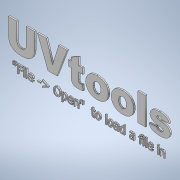
# Autodesk Inventor part: UVtools_demo_file
Saved by Autodesk Inventor 2021 (Build 250183000, 183)
## iProperties
Created: 2020-10-14
Part Number: UVtools_demo_file
Material: Generic
Document SubType Name: Modeling
Designer: tiago
Density: 1 g/cm^3
Appearance: Default
Author: tiago
## iProperties of the stored document _3DPrint.ipt
Created: 2020-10-14
Part Number: _3DPrint
Material: Generic
Document SubType Name: Modeling
Designer: tiago
Density: 1 g/cm^3
Appearance: Default
Author: tiago
Autodesk Inventor part; units mm, degrees
ref_plane "YZ Plane" through (0, 0, 0) normal (1, 0, 0) x (0, 1, 0)
ref_plane "XZ Plane" through (0, 0, 0) normal (0, 1, 0) x (-1, 0, 0)
ref_plane "XY Plane" through (0, 0, 0) normal (0, 0, 1) x (1, 0, 0)
sketch "Sketch1" plane through (0, 0, 0) normal (0, 0, 1) x (1, 0, 0)
  line L0 (-61.4135, 29.5284) -> (63.6527, 29.5284) construction
  line L1 (63.6527, 29.5284) -> (63.6527, 8.7715) construction
  line L2 (63.6527, 8.7715) -> (-61.4135, 8.7715) construction
  line L3 (-61.4135, 8.7715) -> (-61.4135, 29.5284) construction
  line L4 (-61.4135, 8.7715) -> (63.6527, 8.7715) construction
  line L5 (63.6527, 8.7715) -> (63.6527, -11.4157) construction
  line L6 (63.6527, -11.4157) -> (-61.4135, -11.4157) construction
  line L7 (-61.4135, -11.4157) -> (-61.4135, 8.7715) construction
  line L8 (-44.3664, 29.3232) -> (-38.2067, 29.3232)
  line L9 (-38.2067, 29.3232) -> (-38.2067, 17.4079)
  spline S0 degree 2 poles (-38.2067, 17.4079) (-38.2067, 15.6369) (-39.3039, 12.4801) (-41.6716, 10.1316) (-42.9805, 9.6504) knots 0 0 0 1 2 3 3 3
  spline S1 degree 2 poles (-42.9805, 9.6504) (-44.7707, 8.9767) (-47.3116, 8.9767) knots 0 0 0 1 1 1
  spline S2 degree 2 poles (-47.3116, 8.9767) (-48.7745, 8.9767) (-52.2202, 9.3809) (-54.5493, 10.5936) (-56.4742, 12.8265) (-56.8207, 14.02) knots 0 0 0 1 2 3 4 4 4
  spline S3 degree 2 poles (-56.8207, 14.02) (-57.3982, 15.9257) (-57.3982, 17.4079) knots 0 0 0 1 1 1
  line L10 (-57.3982, 17.4079) -> (-57.3982, 29.3232)
  line L11 (-57.3982, 29.3232) -> (-51.2384, 29.3232)
  line L12 (-51.2384, 29.3232) -> (-51.2384, 17.1191)
  spline S4 degree 2 poles (-51.2384, 17.1191) (-51.2384, 15.4829) (-49.4098, 13.635) (-47.7928, 13.635) knots 0 0 0 1 2 2 2
  spline S5 degree 2 poles (-47.7928, 13.635) (-46.1951, 13.635) (-44.3664, 15.4444) (-44.3664, 17.1191) knots 0 0 0 1 2 2 2
  line L13 (-44.3664, 17.1191) -> (-44.3664, 29.3232)
  line L14 (-36.1085, 29.3232) -> (-29.6408, 29.3232)
  line L15 (-29.6408, 29.3232) -> (-25.1172, 14.9247)
  line L16 (-25.1172, 14.9247) -> (-20.6898, 29.3232)
  line L17 (-20.6898, 29.3232) -> (-14.4146, 29.3232)
  line L18 (-14.4146, 29.3232) -> (-21.8448, 9.3232)
  line L19 (-21.8448, 9.3232) -> (-28.5435, 9.3232)
  line L20 (-28.5435, 9.3232) -> (-36.1085, 29.3232)
  line L21 (-6.0411, 29.3232) -> (-6.0411, 23.8179)
  line L22 (-6.0411, 23.8179) -> (-2.9805, 23.8179)
  line L23 (-2.9805, 23.8179) -> (-2.9805, 19.7563)
  line L24 (-2.9805, 19.7563) -> (-6.0411, 19.7563)
  line L25 (-6.0411, 19.7563) -> (-6.0411, 14.6167)
  spline S6 degree 2 poles (-6.0411, 14.6167) (-6.0411, 13.6928) (-5.8679, 13.3848) knots 0 0 0 1 1 1
  spline S7 degree 2 poles (-5.8679, 13.3848) (-5.5984, 12.9228) (-4.9054, 12.9228) knots 0 0 0 1 1 1
  spline S8 degree 2 poles (-4.9054, 12.9228) (-4.2895, 12.9228) (-3.1922, 13.2693) knots 0 0 0 1 1 1
  line L26 (-3.1922, 13.2693) -> (-2.788, 9.4387)
  spline S9 degree 2 poles (-2.788, 9.4387) (-4.8477, 8.9959) (-6.6379, 8.9959) knots 0 0 0 1 1 1
  spline S10 degree 2 poles (-6.6379, 8.9959) (-8.6975, 8.9959) (-10.661, 10.0546) (-11.6042, 12.2298) (-11.6042, 14.6552) knots 0 0 0 1 2 3 3 3
  line L27 (-11.6042, 14.6552) -> (-11.6042, 19.7563)
  line L28 (-11.6042, 19.7563) -> (-13.6446, 19.7563)
  line L29 (-13.6446, 19.7563) -> (-13.6446, 23.8179)
  line L30 (-13.6446, 23.8179) -> (-11.6042, 23.8179)
  line L31 (-11.6042, 23.8179) -> (-11.6042, 26.4743)
  line L32 (-11.6042, 26.4743) -> (-6.0411, 29.3232)
  spline S11 degree 2 poles (-0.9978, 16.5224) (-0.9978, 19.8525) (3.468, 24.1451) (7.2794, 24.1451) knots 0 0 0 1 2 2 2
  spline S12 degree 2 poles (7.2794, 24.1451) (11.6297, 24.1451) (13.8434, 21.6235) knots 0 0 0 1 1 1
  spline S13 degree 2 poles (13.8434, 21.6235) (15.6336, 19.583) (15.6336, 16.6187) knots 0 0 0 1 1 1
  spline S14 degree 2 poles (15.6336, 16.6187) (15.6336, 13.2693) (11.2062, 8.9959) (7.2986, 8.9959) knots 0 0 0 1 2 2 2
  spline S15 degree 2 poles (7.2986, 8.9959) (3.7952, 8.9959) (1.6393, 10.7669) knots 0 0 0 1 1 1
  spline S16 degree 2 poles (1.6393, 10.7669) (-0.9978, 12.9613) (-0.9978, 16.5224) knots 0 0 0 1 1 1
  spline S17 degree 2 poles (4.5652, 16.5417) (4.5652, 14.5975) (6.1244, 12.7495) (7.3179, 12.7495) knots 0 0 0 1 2 2 2
  spline S18 degree 2 poles (7.3179, 12.7495) (8.5113, 12.7495) (10.0513, 14.5782) (10.0513, 16.5994) knots 0 0 0 1 2 2 2
  spline S19 degree 2 poles (10.0513, 16.5994) (10.0513, 18.4666) (8.4921, 20.3145) (7.3564, 20.3145) knots 0 0 0 1 2 2 2
  spline S20 degree 2 poles (7.3564, 20.3145) (6.1437, 20.3145) (4.5652, 18.4473) (4.5652, 16.5417) knots 0 0 0 1 2 2 2
  spline S21 degree 2 poles (17.6547, 16.5224) (17.6547, 19.8525) (22.1206, 24.1451) (25.9319, 24.1451) knots 0 0 0 1 2 2 2
  spline S22 degree 2 poles (25.9319, 24.1451) (30.2823, 24.1451) (32.4959, 21.6235) knots 0 0 0 1 1 1
  spline S23 degree 2 poles (32.4959, 21.6235) (34.2861, 19.583) (34.2861, 16.6187) knots 0 0 0 1 1 1
  spline S24 degree 2 poles (34.2861, 16.6187) (34.2861, 13.2693) (29.8588, 8.9959) (25.9512, 8.9959) knots 0 0 0 1 2 2 2
  spline S25 degree 2 poles (25.9512, 8.9959) (22.4478, 8.9959) (20.2919, 10.7669) knots 0 0 0 1 1 1
  spline S26 degree 2 poles (20.2919, 10.7669) (17.6547, 12.9613) (17.6547, 16.5224) knots 0 0 0 1 1 1
  spline S27 degree 2 poles (23.2178, 16.5417) (23.2178, 14.5975) (24.777, 12.7495) (25.9704, 12.7495) knots 0 0 0 1 2 2 2
  spline S28 degree 2 poles (25.9704, 12.7495) (27.1639, 12.7495) (28.7038, 14.5782) (28.7038, 16.5994) knots 0 0 0 1 2 2 2
  spline S29 degree 2 poles (28.7038, 16.5994) (28.7038, 18.4666) (27.1446, 20.3145) (26.0089, 20.3145) knots 0 0 0 1 2 2 2
  spline S30 degree 2 poles (26.0089, 20.3145) (24.7962, 20.3145) (23.2178, 18.4473) (23.2178, 16.5417) knots 0 0 0 1 2 2 2
  line L33 (37.1735, 29.3232) -> (42.7365, 29.3232)
  line L34 (42.7365, 29.3232) -> (42.7365, 9.3232)
  line L35 (42.7365, 9.3232) -> (37.1735, 9.3232)
  line L36 (37.1735, 9.3232) -> (37.1735, 29.3232)
  line L37 (45.3159, 13.3463) -> (50.8212, 13.866)
  spline S31 degree 2 poles (50.8212, 13.866) (51.1677, 12.8843) (52.3997, 12.0373) (53.4199, 12.0373) knots 0 0 0 1 2 2 2
  spline S32 degree 2 poles (53.4199, 12.0373) (54.5556, 12.0373) (55.1716, 12.5186) knots 0 0 0 1 1 1
  spline S33 degree 2 poles (55.1716, 12.5186) (55.6528, 12.865) (55.6528, 13.404) knots 0 0 0 1 1 1
  spline S34 degree 2 poles (55.6528, 13.404) (55.6528, 14.0008) (55.0176, 14.328) knots 0 0 0 1 1 1
  spline S35 degree 2 poles (55.0176, 14.328) (54.5556, 14.559) (52.6307, 14.9055) knots 0 0 0 1 1 1
  spline S36 degree 2 poles (52.6307, 14.9055) (49.724, 15.4059) (47.4719, 16.2722) (45.9319, 18.3126) (45.9319, 19.6215) knots 0 0 0 1 2 3 3 3
  spline S37 degree 2 poles (45.9319, 19.6215) (45.9319, 21.046) (47.6066, 23.1249) (50.5132, 24.1451) (52.9772, 24.1451) knots 0 0 0 1 2 3 3 3
  spline S38 degree 2 poles (52.9772, 24.1451) (55.5758, 24.1451) (58.0397, 23.3559) (59.6951, 21.7005) (60.2341, 20.276) knots 0 0 0 1 2 3 3 3
  line L38 (60.2341, 20.276) -> (54.9598, 19.7563)
  spline S39 degree 2 poles (54.9598, 19.7563) (54.7481, 20.4493) (54.2861, 20.7765) knots 0 0 0 1 1 1
  spline S40 degree 2 poles (54.2861, 20.7765) (53.6316, 21.2192) (52.6884, 21.2192) knots 0 0 0 1 1 1
  spline S41 degree 2 poles (52.6884, 21.2192) (51.7644, 21.2192) (50.8982, 20.5455) (50.8982, 20.0643) knots 0 0 0 1 2 2 2
  spline S42 degree 2 poles (50.8982, 20.0643) (50.8982, 19.5445) (51.4565, 19.2751) knots 0 0 0 1 1 1
  spline S43 degree 2 poles (51.4565, 19.2751) (51.9954, 18.9863) (53.8241, 18.7746) knots 0 0 0 1 1 1
  spline S44 degree 2 poles (53.8241, 18.7746) (56.596, 18.4666) (59.3102, 17.3501) (60.7346, 15.2712) (60.7346, 14.0392) knots 0 0 0 1 2 3 3 3
  spline S45 degree 2 poles (60.7346, 14.0392) (60.7346, 12.7688) (59.2139, 10.4011) (55.9608, 8.9959) (53.1504, 8.9959) knots 0 0 0 1 2 3 3 3
  spline S46 degree 2 poles (53.1504, 8.9959) (49.1658, 8.9959) (45.7972, 11.2674) (45.3159, 13.3463) knots 0 0 0 1 2 2 2
  line L39 (-52.0538, 2.6212) -> (-52.2289, 0.2873)
  line L40 (-52.2289, 0.2873) -> (-52.7589, 0.2873)
  line L41 (-52.7589, 0.2873) -> (-52.9339, 2.6212)
  line L42 (-52.9339, 2.6212) -> (-52.0538, 2.6212)
  line L43 (-53.5708, 2.6212) -> (-53.7459, 0.2873)
  line L44 (-53.7459, 0.2873) -> (-54.2759, 0.2873)
  line L45 (-54.2759, 0.2873) -> (-54.4509, 2.6212)
  line L46 (-54.4509, 2.6212) -> (-53.5708, 2.6212)
  line L47 (-47.4007, 1.6438) -> (-50.1916, 1.6438)
  line L48 (-50.1916, 1.6438) -> (-50.1916, -0.0482)
  line L49 (-50.1916, -0.0482) -> (-47.5174, -0.0482)
  line L50 (-47.5174, -0.0482) -> (-47.5174, -0.7581)
  line L51 (-47.5174, -0.7581) -> (-50.1916, -0.7581)
  line L52 (-50.1916, -0.7581) -> (-50.1916, -3.6463)
  line L53 (-50.1916, -3.6463) -> (-50.989, -3.6463)
  line L54 (-50.989, -3.6463) -> (-50.989, 2.3537)
  line L55 (-50.989, 2.3537) -> (-47.4007, 2.3537)
  line L56 (-47.4007, 2.3537) -> (-47.4007, 1.6438)
  line L57 (-45.9712, -3.6463) -> (-46.7297, -3.6463)
  line L58 (-46.7297, -3.6463) -> (-46.7297, 0.8562)
  line L59 (-46.7297, 0.8562) -> (-45.9712, 0.8562)
  line L60 (-45.9712, 0.8562) -> (-45.9712, -3.6463)
  line L61 (-45.9177, 1.6049) -> (-46.7783, 1.6049)
  line L62 (-46.7783, 1.6049) -> (-46.7783, 2.3926)
  line L63 (-46.7783, 2.3926) -> (-45.9177, 2.3926)
  line L64 (-45.9177, 2.3926) -> (-45.9177, 1.6049)
  line L65 (-44.0846, -3.6463) -> (-44.8431, -3.6463)
  line L66 (-44.8431, -3.6463) -> (-44.8431, 2.6212)
  line L67 (-44.8431, 2.6212) -> (-44.0846, 2.6212)
  line L68 (-44.0846, 2.6212) -> (-44.0846, -3.6463)
  spline S47 degree 2 poles (-41.0165, -3.7484) (-42.096, -3.7484) (-43.2824, -2.5377) (-43.2824, -1.4194) knots 0 0 0 1 2 2 2
  spline S48 degree 2 poles (-43.2824, -1.4194) (-43.2824, -0.3205) (-42.13, 0.9826) (-41.2013, 0.9826) knots 0 0 0 1 2 2 2
  spline S49 degree 2 poles (-41.2013, 0.9826) (-40.7832, 0.9826) (-40.1365, 0.7395) (-39.8982, 0.4818) knots 0 0 0 1 2 2 2
  spline S50 degree 2 poles (-39.8982, 0.4818) (-39.6551, 0.2241) (-39.3974, -0.5199) (-39.3974, -1.0596) knots 0 0 0 1 2 2 2
  line L69 (-39.3974, -1.0596) -> (-39.3974, -1.4729)
  line L70 (-39.3974, -1.4729) -> (-42.5141, -1.4729)
  spline S51 degree 2 poles (-42.5141, -1.4729) (-42.5141, -2.2557) (-41.7264, -3.0871) (-41.0263, -3.0871) knots 0 0 0 1 2 2 2
  spline S52 degree 2 poles (-41.0263, -3.0871) (-40.7783, -3.0871) (-40.2969, -2.9753) (-40.1024, -2.8878) knots 0 0 0 1 2 2 2
  spline S53 degree 2 poles (-40.1024, -2.8878) (-39.8982, -2.7905) (-39.6162, -2.6203) (-39.5238, -2.5425) knots 0 0 0 1 2 2 2
  line L71 (-39.5238, -2.5425) -> (-39.4801, -2.5425)
  line L72 (-39.4801, -2.5425) -> (-39.4801, -3.3691)
  spline S54 degree 2 poles (-39.4801, -3.3691) (-39.6114, -3.4226) (-40.0101, -3.5782) (-40.1657, -3.622) knots 0 0 0 1 2 2 2
  spline S55 degree 2 poles (-40.1657, -3.622) (-40.3845, -3.6852) (-40.7443, -3.7484) (-41.0165, -3.7484) knots 0 0 0 1 2 2 2
  spline S56 degree 2 poles (-40.1365, -0.8942) (-40.1462, -0.5879) (-40.2726, -0.1406) (-40.3942, 0.0101) knots 0 0 0 1 2 2 2
  spline S57 degree 2 poles (-40.3942, 0.0101) (-40.5255, 0.1803) (-40.9388, 0.3602) (-41.2451, 0.3602) knots 0 0 0 1 2 2 2
  spline S58 degree 2 poles (-41.2451, 0.3602) (-41.5465, 0.3602) (-41.9695, 0.1803) (-42.1446, 0.0053) knots 0 0 0 1 2 2 2
  spline S59 degree 2 poles (-42.1446, 0.0053) (-42.3148, -0.1746) (-42.4898, -0.6074) (-42.5141, -0.8942) knots 0 0 0 1 2 2 2
  line L73 (-42.5141, -0.8942) -> (-40.1365, -0.8942)
  line L74 (-33.9663, -1.3853) -> (-36.237, -1.3853)
  line L75 (-36.237, -1.3853) -> (-36.237, -0.656)
  line L76 (-36.237, -0.656) -> (-33.9663, -0.656)
  line L77 (-33.9663, -0.656) -> (-33.9663, -1.3853)
  line L78 (-28.4136, -1.2638) -> (-32.741, -3.3302)
  line L79 (-32.741, -3.3302) -> (-32.741, -2.6155)
  line L80 (-32.741, -2.6155) -> (-29.3861, -1.0207)
  line L81 (-29.3861, -1.0207) -> (-32.741, 0.5693)
  line L82 (-32.741, 0.5693) -> (-32.741, 1.284)
  line L83 (-32.741, 1.284) -> (-28.4136, -0.7824)
  line L84 (-28.4136, -0.7824) -> (-28.4136, -1.2638)
  spline S60 degree 2 poles (-20.1721, 1.6682) (-19.8318, 1.2694) (-19.4525, 0.1025) (-19.4525, -0.6463) knots 0 0 0 1 2 2 2
  spline S61 degree 2 poles (-19.4525, -0.6463) (-19.4525, -1.3756) (-19.8221, -2.5571) (-20.1721, -2.9558) knots 0 0 0 1 2 2 2
  spline S62 degree 2 poles (-20.1721, -2.9558) (-20.5417, -3.374) (-21.519, -3.7727) (-22.1073, -3.7727) knots 0 0 0 1 2 2 2
  spline S63 degree 2 poles (-22.1073, -3.7727) (-22.7151, -3.7727) (-23.6875, -3.3594) (-24.0425, -2.9558) knots 0 0 0 1 2 2 2
  spline S64 degree 2 poles (-24.0425, -2.9558) (-24.3877, -2.5571) (-24.7572, -1.3853) (-24.7572, -0.6463) knots 0 0 0 1 2 2 2
  spline S65 degree 2 poles (-24.7572, -0.6463) (-24.7572, 0.1074) (-24.3828, 1.2549) (-24.0376, 1.6682) knots 0 0 0 1 2 2 2
  spline S66 degree 2 poles (-24.0376, 1.6682) (-23.6875, 2.0669) (-22.7102, 2.4801) (-22.1073, 2.4801) knots 0 0 0 1 2 2 2
  spline S67 degree 2 poles (-22.1073, 2.4801) (-21.4947, 2.4801) (-20.5125, 2.0523) (-20.1721, 1.6682) knots 0 0 0 1 2 2 2
  spline S68 degree 2 poles (-20.284, -0.6463) (-20.284, -0.0531) (-20.5417, 0.8659) (-20.7751, 1.1673) knots 0 0 0 1 2 2 2
  spline S69 degree 2 poles (-20.7751, 1.1673) (-21.0133, 1.4785) (-21.6843, 1.7897) (-22.1024, 1.7897) knots 0 0 0 1 2 2 2
  spline S70 degree 2 poles (-22.1024, 1.7897) (-22.5352, 1.7897) (-23.1867, 1.4882) (-23.4347, 1.1673) knots 0 0 0 1 2 2 2
  spline S71 degree 2 poles (-23.4347, 1.1673) (-23.673, 0.861) (-23.9258, -0.0628) (-23.9258, -0.6463) knots 0 0 0 1 2 2 2
  spline S72 degree 2 poles (-23.9258, -0.6463) (-23.9258, -1.8278) (-22.9339, -3.0823) (-22.1024, -3.0823) knots 0 0 0 1 2 2 2
  spline S73 degree 2 poles (-22.1024, -3.0823) (-21.271, -3.0823) (-20.284, -1.8278) (-20.284, -0.6463) knots 0 0 0 1 2 2 2
  spline S74 degree 2 poles (-14.8626, -1.2735) (-14.8626, -2.4015) (-15.9371, -3.7338) (-16.7589, -3.7338) knots 0 0 0 1 2 2 2
  spline S75 degree 2 poles (-16.7589, -3.7338) (-17.0943, -3.7338) (-17.6097, -3.5782) (-17.8772, -3.4177) knots 0 0 0 1 2 2 2
  line L85 (-17.8772, -3.4177) -> (-17.8772, -5.3043)
  line L86 (-17.8772, -5.3043) -> (-18.6357, -5.3043)
  line L87 (-18.6357, -5.3043) -> (-18.6357, 0.8562)
  line L88 (-18.6357, 0.8562) -> (-17.8772, 0.8562)
  line L89 (-17.8772, 0.8562) -> (-17.8772, 0.3845)
  spline S76 degree 2 poles (-17.8772, 0.3845) (-17.5952, 0.6422) (-16.9047, 0.9826) (-16.5012, 0.9826) knots 0 0 0 1 2 2 2
  spline S77 degree 2 poles (-16.5012, 0.9826) (-15.7281, 0.9826) (-14.8626, -0.2427) (-14.8626, -1.2735) knots 0 0 0 1 2 2 2
  spline S78 degree 2 poles (-15.6454, -1.361) (-15.6454, -0.5879) (-16.1365, 0.263) (-16.6859, 0.263) knots 0 0 0 1 2 2 2
  spline S79 degree 2 poles (-16.6859, 0.263) (-17.0068, 0.263) (-17.6097, -0.0239) (-17.8772, -0.2476) knots 0 0 0 1 2 2 2
  line L90 (-17.8772, -0.2476) -> (-17.8772, -2.8051)
  spline S80 degree 2 poles (-17.8772, -2.8051) (-17.5806, -2.9461) (-17.1576, -3.0531) (-16.8853, -3.0531) knots 0 0 0 1 2 2 2
  spline S81 degree 2 poles (-16.8853, -3.0531) (-16.2969, -3.0531) (-15.6454, -2.1876) (-15.6454, -1.361) knots 0 0 0 1 2 2 2
  spline S82 degree 2 poles (-12.1203, -3.7484) (-13.1997, -3.7484) (-14.3861, -2.5377) (-14.3861, -1.4194) knots 0 0 0 1 2 2 2
  spline S83 degree 2 poles (-14.3861, -1.4194) (-14.3861, -0.3205) (-13.2337, 0.9826) (-12.305, 0.9826) knots 0 0 0 1 2 2 2
  spline S84 degree 2 poles (-12.305, 0.9826) (-11.8869, 0.9826) (-11.2402, 0.7395) (-11.002, 0.4818) knots 0 0 0 1 2 2 2
  spline S85 degree 2 poles (-11.002, 0.4818) (-10.7588, 0.2241) (-10.5012, -0.5199) (-10.5012, -1.0596) knots 0 0 0 1 2 2 2
  line L91 (-10.5012, -1.0596) -> (-10.5012, -1.4729)
  line L92 (-10.5012, -1.4729) -> (-13.6178, -1.4729)
  spline S86 degree 2 poles (-13.6178, -1.4729) (-13.6178, -2.2557) (-12.8302, -3.0871) (-12.13, -3.0871) knots 0 0 0 1 2 2 2
  spline S87 degree 2 poles (-12.13, -3.0871) (-11.882, -3.0871) (-11.4007, -2.9753) (-11.2062, -2.8878) knots 0 0 0 1 2 2 2
  spline S88 degree 2 poles (-11.2062, -2.8878) (-11.002, -2.7905) (-10.72, -2.6203) (-10.6276, -2.5425) knots 0 0 0 1 2 2 2
  line L93 (-10.6276, -2.5425) -> (-10.5838, -2.5425)
  line L94 (-10.5838, -2.5425) -> (-10.5838, -3.3691)
  spline S89 degree 2 poles (-10.5838, -3.3691) (-10.7151, -3.4226) (-11.1138, -3.5782) (-11.2694, -3.622) knots 0 0 0 1 2 2 2
  spline S90 degree 2 poles (-11.2694, -3.622) (-11.4882, -3.6852) (-11.848, -3.7484) (-12.1203, -3.7484) knots 0 0 0 1 2 2 2
  spline S91 degree 2 poles (-11.2402, -0.8942) (-11.2499, -0.5879) (-11.3764, -0.1406) (-11.4979, 0.0101) knots 0 0 0 1 2 2 2
  spline S92 degree 2 poles (-11.4979, 0.0101) (-11.6292, 0.1803) (-12.0425, 0.3602) (-12.3488, 0.3602) knots 0 0 0 1 2 2 2
  spline S93 degree 2 poles (-12.3488, 0.3602) (-12.6503, 0.3602) (-13.0733, 0.1803) (-13.2483, 0.0053) knots 0 0 0 1 2 2 2
  spline S94 degree 2 poles (-13.2483, 0.0053) (-13.4185, -0.1746) (-13.5935, -0.6074) (-13.6178, -0.8942) knots 0 0 0 1 2 2 2
  line L95 (-13.6178, -0.8942) -> (-11.2402, -0.8942)
  line L96 (-6.1981, -3.6463) -> (-6.9566, -3.6463)
  line L97 (-6.9566, -3.6463) -> (-6.9566, -1.079)
  spline S95 degree 2 poles (-6.9566, -1.079) (-6.9566, -0.7678) (-7.0149, -0.233) (-7.1024, -0.0725) knots 0 0 0 1 2 2 2
  spline S96 degree 2 poles (-7.1024, -0.0725) (-7.1948, 0.0976) (-7.5255, 0.263) (-7.8075, 0.263) knots 0 0 0 1 2 2 2
  spline S97 degree 2 poles (-7.8075, 0.263) (-8.0895, 0.263) (-8.6875, -0.0385) (-8.9744, -0.2816) knots 0 0 0 1 2 2 2
  line L98 (-8.9744, -0.2816) -> (-8.9744, -3.6463)
  line L99 (-8.9744, -3.6463) -> (-9.7329, -3.6463)
  line L100 (-9.7329, -3.6463) -> (-9.7329, 0.8562)
  line L101 (-9.7329, 0.8562) -> (-8.9744, 0.8562)
  line L102 (-8.9744, 0.8562) -> (-8.9744, 0.3553)
  spline S98 degree 2 poles (-8.9744, 0.3553) (-8.6341, 0.6617) (-7.9777, 0.9826) (-7.6081, 0.9826) knots 0 0 0 1 2 2 2
  spline S99 degree 2 poles (-7.6081, 0.9826) (-6.9469, 0.9826) (-6.1981, 0.1074) (-6.1981, -0.7241) knots 0 0 0 1 2 2 2
  line L103 (-6.1981, -0.7241) -> (-6.1981, -3.6463)
  line L104 (-4.3456, 2.6212) -> (-4.5206, 0.2873)
  line L105 (-4.5206, 0.2873) -> (-5.0506, 0.2873)
  line L106 (-5.0506, 0.2873) -> (-5.2256, 2.6212)
  line L107 (-5.2256, 2.6212) -> (-4.3456, 2.6212)
  line L108 (-2.8285, 2.6212) -> (-3.0036, 0.2873)
  line L109 (-3.0036, 0.2873) -> (-3.5336, 0.2873)
  line L110 (-3.5336, 0.2873) -> (-3.7086, 2.6212)
  line L111 (-3.7086, 2.6212) -> (-2.8285, 2.6212)
  spline S100 degree 2 poles (4.6933, -3.7338) (4.0758, -3.7338) (3.3805, -3.0288) (3.3805, -2.2654) knots 0 0 0 1 2 2 2
  line L112 (3.3805, -2.2654) -> (3.3805, 0.2289)
  line L113 (3.3805, 0.2289) -> (2.87, 0.2289)
  line L114 (2.87, 0.2289) -> (2.87, 0.8562)
  line L115 (2.87, 0.8562) -> (3.3805, 0.8562)
  line L116 (3.3805, 0.8562) -> (3.3805, 2.1495)
  line L117 (3.3805, 2.1495) -> (4.139, 2.1495)
  line L118 (4.139, 2.1495) -> (4.139, 0.8562)
  line L119 (4.139, 0.8562) -> (5.5345, 0.8562)
  line L120 (5.5345, 0.8562) -> (5.5345, 0.2289)
  line L121 (5.5345, 0.2289) -> (4.139, 0.2289)
  line L122 (4.139, 0.2289) -> (4.139, -1.9153)
  spline S101 degree 2 poles (4.139, -1.9153) (4.139, -2.2557) (4.1634, -2.6301) (4.246, -2.7905) knots 0 0 0 1 2 2 2
  spline S102 degree 2 poles (4.246, -2.7905) (4.3141, -2.9315) (4.6204, -3.0725) (4.883, -3.0725) knots 0 0 0 1 2 2 2
  spline S103 degree 2 poles (4.883, -3.0725) (5.0677, -3.0725) (5.4129, -2.9607) (5.4907, -2.9267) knots 0 0 0 1 2 2 2
  line L123 (5.4907, -2.9267) -> (5.5345, -2.9267)
  line L124 (5.5345, -2.9267) -> (5.5345, -3.6074)
  spline S104 degree 2 poles (5.5345, -3.6074) (5.3206, -3.6657) (4.883, -3.7338) (4.6933, -3.7338) knots 0 0 0 1 2 2 2
  spline S105 degree 2 poles (9.7938, -1.3951) (9.7938, -2.5328) (8.6998, -3.7727) (7.7857, -3.7727) knots 0 0 0 1 2 2 2
  spline S106 degree 2 poles (7.7857, -3.7727) (6.8473, -3.7727) (5.7728, -2.4939) (5.7728, -1.3951) knots 0 0 0 1 2 2 2
  spline S107 degree 2 poles (5.7728, -1.3951) (5.7728, -0.267) (6.8813, 0.9826) (7.7857, 0.9826) knots 0 0 0 1 2 2 2
  spline S108 degree 2 poles (7.7857, 0.9826) (8.6998, 0.9826) (9.7938, -0.2622) (9.7938, -1.3951) knots 0 0 0 1 2 2 2
  spline S109 degree 2 poles (9.011, -1.3951) (9.011, -0.5199) (8.3741, 0.331) (7.7857, 0.331) knots 0 0 0 1 2 2 2
  spline S110 degree 2 poles (7.7857, 0.331) (7.1974, 0.331) (6.5556, -0.5199) (6.5556, -1.3951) knots 0 0 0 1 2 2 2
  spline S111 degree 2 poles (6.5556, -1.3951) (6.5556, -2.2459) (7.1974, -3.1212) (7.7857, -3.1212) knots 0 0 0 1 2 2 2
  spline S112 degree 2 poles (7.7857, -3.1212) (8.3692, -3.1212) (9.011, -2.2605) (9.011, -1.3951) knots 0 0 0 1 2 2 2
  line L125 (13.9219, -3.6463) -> (13.1634, -3.6463)
  line L126 (13.1634, -3.6463) -> (13.1634, 2.6212)
  line L127 (13.1634, 2.6212) -> (13.9219, 2.6212)
  line L128 (13.9219, 2.6212) -> (13.9219, -3.6463)
  spline S113 degree 2 poles (18.7355, -1.3951) (18.7355, -2.5328) (17.6415, -3.7727) (16.7274, -3.7727) knots 0 0 0 1 2 2 2
  spline S114 degree 2 poles (16.7274, -3.7727) (15.789, -3.7727) (14.7144, -2.4939) (14.7144, -1.3951) knots 0 0 0 1 2 2 2
  spline S115 degree 2 poles (14.7144, -1.3951) (14.7144, -0.267) (15.823, 0.9826) (16.7274, 0.9826) knots 0 0 0 1 2 2 2
  spline S116 degree 2 poles (16.7274, 0.9826) (17.6415, 0.9826) (18.7355, -0.2622) (18.7355, -1.3951) knots 0 0 0 1 2 2 2
  spline S117 degree 2 poles (17.9527, -1.3951) (17.9527, -0.5199) (17.3157, 0.331) (16.7274, 0.331) knots 0 0 0 1 2 2 2
  spline S118 degree 2 poles (16.7274, 0.331) (16.139, 0.331) (15.4972, -0.5199) (15.4972, -1.3951) knots 0 0 0 1 2 2 2
  spline S119 degree 2 poles (15.4972, -1.3951) (15.4972, -2.2459) (16.139, -3.1212) (16.7274, -3.1212) knots 0 0 0 1 2 2 2
  spline S120 degree 2 poles (16.7274, -3.1212) (17.3108, -3.1212) (17.9527, -2.2605) (17.9527, -1.3951) knots 0 0 0 1 2 2 2
  spline S121 degree 2 poles (22.0224, -3.1698) (21.93, -3.2378) (21.6188, -3.481) (21.4729, -3.5539) knots 0 0 0 1 2 2 2
  spline S122 degree 2 poles (21.4729, -3.5539) (21.2736, -3.6609) (20.8992, -3.7727) (20.5588, -3.7727) knots 0 0 0 1 2 2 2
  spline S123 degree 2 poles (20.5588, -3.7727) (20.2817, -3.7727) (19.7809, -3.5636) (19.5912, -3.374) knots 0 0 0 1 2 2 2
  spline S124 degree 2 poles (19.5912, -3.374) (19.4113, -3.1892) (19.1925, -2.6447) (19.1925, -2.3432) knots 0 0 0 1 2 2 2
  spline S125 degree 2 poles (19.1925, -2.3432) (19.1925, -1.8764) (19.5864, -1.2152) (20.0142, -1.0255) knots 0 0 0 1 2 2 2
  spline S126 degree 2 poles (20.0142, -1.0255) (20.3935, -0.8505) (21.4243, -0.7192) (22.0224, -0.6852) knots 0 0 0 1 2 2 2
  line L129 (22.0224, -0.6852) -> (22.0224, -0.5393)
  spline S127 degree 2 poles (22.0224, -0.5393) (22.0224, -0.2767) (21.8619, 0.049) (21.716, 0.1414) knots 0 0 0 1 2 2 2
  spline S128 degree 2 poles (21.716, 0.1414) (21.5702, 0.2338) (21.152, 0.2921) (20.9283, 0.2921) knots 0 0 0 1 2 2 2
  spline S129 degree 2 poles (20.9283, 0.2921) (20.6658, 0.2921) (19.9559, 0.1365) (19.601, -0.0142) knots 0 0 0 1 2 2 2
  line L130 (19.601, -0.0142) -> (19.5572, -0.0142)
  line L131 (19.5572, -0.0142) -> (19.5572, 0.7589)
  spline S130 degree 2 poles (19.5572, 0.7589) (19.7663, 0.8173) (20.5491, 0.9631) (20.9332, 0.9631) knots 0 0 0 1 2 2 2
  spline S131 degree 2 poles (20.9332, 0.9631) (21.4, 0.9631) (22.0369, 0.8173) (22.2898, 0.6276) knots 0 0 0 1 2 2 2
  spline S132 degree 2 poles (22.2898, 0.6276) (22.5377, 0.4429) (22.7809, -0.1455) (22.7809, -0.5685) knots 0 0 0 1 2 2 2
  line L132 (22.7809, -0.5685) -> (22.7809, -3.6463)
  line L133 (22.7809, -3.6463) -> (22.0224, -3.6463)
  line L134 (22.0224, -3.6463) -> (22.0224, -3.1698)
  line L135 (22.0224, -2.5377) -> (22.0224, -1.2881)
  spline S133 degree 2 poles (22.0224, -1.2881) (21.7501, -1.3124) (20.9283, -1.3951) (20.6706, -1.4729) knots 0 0 0 1 2 2 2
  spline S134 degree 2 poles (20.6706, -1.4729) (20.3692, -1.5652) (19.9753, -1.9494) (19.9753, -2.2897) knots 0 0 0 1 2 2 2
  spline S135 degree 2 poles (19.9753, -2.2897) (19.9753, -2.6787) (20.413, -3.0725) (20.8311, -3.0725) knots 0 0 0 1 2 2 2
  spline S136 degree 2 poles (20.8311, -3.0725) (21.186, -3.0725) (21.7695, -2.7662) (22.0224, -2.5377) knots 0 0 0 1 2 2 2
  line L136 (27.3076, -3.6463) -> (26.5491, -3.6463)
  line L137 (26.5491, -3.6463) -> (26.5491, -3.1892)
  spline S137 degree 2 poles (26.5491, -3.1892) (26.3741, -3.3351) (26.1164, -3.5296) (25.9413, -3.6122) knots 0 0 0 1 2 2 2
  spline S138 degree 2 poles (25.9413, -3.6122) (25.7809, -3.69) (25.4356, -3.7727) (25.2071, -3.7727) knots 0 0 0 1 2 2 2
  spline S139 degree 2 poles (25.2071, -3.7727) (24.8376, -3.7727) (24.2152, -3.4664) (23.9964, -3.1698) knots 0 0 0 1 2 2 2
  spline S140 degree 2 poles (23.9964, -3.1698) (23.7776, -2.8732) (23.5345, -1.998) (23.5345, -1.4291) knots 0 0 0 1 2 2 2
  spline S141 degree 2 poles (23.5345, -1.4291) (23.5345, -0.8359) (23.8408, 0.0296) (24.1083, 0.3553) knots 0 0 0 1 2 2 2
  spline S142 degree 2 poles (24.1083, 0.3553) (24.3562, 0.6471) (25.0515, 0.9826) (25.4356, 0.9826) knots 0 0 0 1 2 2 2
  spline S143 degree 2 poles (25.4356, 0.9826) (25.7711, 0.9826) (26.2719, 0.8318) (26.5491, 0.6763) knots 0 0 0 1 2 2 2
  line L138 (26.5491, 0.6763) -> (26.5491, 2.6212)
  line L139 (26.5491, 2.6212) -> (27.3076, 2.6212)
  line L140 (27.3076, 2.6212) -> (27.3076, -3.6463)
  line L141 (26.5491, -2.5523) -> (26.5491, 0.049)
  spline S144 degree 2 poles (26.5491, 0.049) (26.2671, 0.1852) (25.8198, 0.2873) (25.5621, 0.2873) knots 0 0 0 1 2 2 2
  spline S145 degree 2 poles (25.5621, 0.2873) (24.9786, 0.2873) (24.3173, -0.5879) (24.3173, -1.4145) knots 0 0 0 1 2 2 2
  spline S146 degree 2 poles (24.3173, -1.4145) (24.3173, -2.2119) (24.823, -3.0531) (25.3822, -3.0531) knots 0 0 0 1 2 2 2
  spline S147 degree 2 poles (25.3822, -3.0531) (25.6788, -3.0531) (26.2817, -2.7808) (26.5491, -2.5523) knots 0 0 0 1 2 2 2
  spline S148 degree 2 poles (33.4924, -3.1698) (33.4, -3.2378) (33.0888, -3.481) (32.9429, -3.5539) knots 0 0 0 1 2 2 2
  spline S149 degree 2 poles (32.9429, -3.5539) (32.7436, -3.6609) (32.3692, -3.7727) (32.0288, -3.7727) knots 0 0 0 1 2 2 2
  spline S150 degree 2 poles (32.0288, -3.7727) (31.7517, -3.7727) (31.2509, -3.5636) (31.0612, -3.374) knots 0 0 0 1 2 2 2
  spline S151 degree 2 poles (31.0612, -3.374) (30.8813, -3.1892) (30.6625, -2.6447) (30.6625, -2.3432) knots 0 0 0 1 2 2 2
  spline S152 degree 2 poles (30.6625, -2.3432) (30.6625, -1.8764) (31.0564, -1.2152) (31.4843, -1.0255) knots 0 0 0 1 2 2 2
  spline S153 degree 2 poles (31.4843, -1.0255) (31.8635, -0.8505) (32.8943, -0.7192) (33.4924, -0.6852) knots 0 0 0 1 2 2 2
  line L142 (33.4924, -0.6852) -> (33.4924, -0.5393)
  spline S154 degree 2 poles (33.4924, -0.5393) (33.4924, -0.2767) (33.3319, 0.049) (33.186, 0.1414) knots 0 0 0 1 2 2 2
  spline S155 degree 2 poles (33.186, 0.1414) (33.0402, 0.2338) (32.622, 0.2921) (32.3984, 0.2921) knots 0 0 0 1 2 2 2
  spline S156 degree 2 poles (32.3984, 0.2921) (32.1358, 0.2921) (31.4259, 0.1365) (31.071, -0.0142) knots 0 0 0 1 2 2 2
  line L143 (31.071, -0.0142) -> (31.0272, -0.0142)
  line L144 (31.0272, -0.0142) -> (31.0272, 0.7589)
  spline S157 degree 2 poles (31.0272, 0.7589) (31.2363, 0.8173) (32.0191, 0.9631) (32.4032, 0.9631) knots 0 0 0 1 2 2 2
  spline S158 degree 2 poles (32.4032, 0.9631) (32.87, 0.9631) (33.507, 0.8173) (33.7598, 0.6276) knots 0 0 0 1 2 2 2
  spline S159 degree 2 poles (33.7598, 0.6276) (34.0078, 0.4429) (34.2509, -0.1455) (34.2509, -0.5685) knots 0 0 0 1 2 2 2
  line L145 (34.2509, -0.5685) -> (34.2509, -3.6463)
  line L146 (34.2509, -3.6463) -> (33.4924, -3.6463)
  line L147 (33.4924, -3.6463) -> (33.4924, -3.1698)
  line L148 (33.4924, -2.5377) -> (33.4924, -1.2881)
  spline S160 degree 2 poles (33.4924, -1.2881) (33.2201, -1.3124) (32.3984, -1.3951) (32.1407, -1.4729) knots 0 0 0 1 2 2 2
  spline S161 degree 2 poles (32.1407, -1.4729) (31.8392, -1.5652) (31.4454, -1.9494) (31.4454, -2.2897) knots 0 0 0 1 2 2 2
  spline S162 degree 2 poles (31.4454, -2.2897) (31.4454, -2.6787) (31.883, -3.0725) (32.3011, -3.0725) knots 0 0 0 1 2 2 2
  spline S163 degree 2 poles (32.3011, -3.0725) (32.6561, -3.0725) (33.2395, -2.7662) (33.4924, -2.5377) knots 0 0 0 1 2 2 2
  line L149 (40.2606, 1.8918) -> (40.2217, 1.8918)
  spline S164 degree 2 poles (40.2217, 1.8918) (40.1196, 1.9307) (39.7403, 1.9988) (39.5896, 1.9988) knots 0 0 0 1 2 2 2
  spline S165 degree 2 poles (39.5896, 1.9988) (39.1131, 1.9988) (38.7047, 1.5709) (38.7047, 1.0069) knots 0 0 0 1 2 2 2
  line L150 (38.7047, 1.0069) -> (38.7047, 0.8562)
  line L151 (38.7047, 0.8562) -> (39.9591, 0.8562)
  line L152 (39.9591, 0.8562) -> (39.9591, 0.2289)
  line L153 (39.9591, 0.2289) -> (38.729, 0.2289)
  line L154 (38.729, 0.2289) -> (38.729, -3.6463)
  line L155 (38.729, -3.6463) -> (37.9705, -3.6463)
  line L156 (37.9705, -3.6463) -> (37.9705, 0.2289)
  line L157 (37.9705, 0.2289) -> (37.46, 0.2289)
  line L158 (37.46, 0.2289) -> (37.46, 0.8562)
  line L159 (37.46, 0.8562) -> (37.9705, 0.8562)
  line L160 (37.9705, 0.8562) -> (37.9705, 1.0069)
  spline S166 degree 2 poles (37.9705, 1.0069) (37.9705, 1.814) (38.7533, 2.66) (39.4826, 2.66) knots 0 0 0 1 2 2 2
  spline S167 degree 2 poles (39.4826, 2.66) (39.6917, 2.66) (40.0953, 2.6163) (40.2606, 2.5871) knots 0 0 0 1 2 2 2
  line L161 (40.2606, 2.5871) -> (40.2606, 1.8918)
  line L162 (41.2914, -3.6463) -> (40.5329, -3.6463)
  line L163 (40.5329, -3.6463) -> (40.5329, 0.8562)
  line L164 (40.5329, 0.8562) -> (41.2914, 0.8562)
  line L165 (41.2914, 0.8562) -> (41.2914, -3.6463)
  line L166 (41.3449, 1.6049) -> (40.4843, 1.6049)
  line L167 (40.4843, 1.6049) -> (40.4843, 2.3926)
  line L168 (40.4843, 2.3926) -> (41.3449, 2.3926)
  line L169 (41.3449, 2.3926) -> (41.3449, 1.6049)
  line L170 (43.1779, -3.6463) -> (42.4194, -3.6463)
  line L171 (42.4194, -3.6463) -> (42.4194, 2.6212)
  line L172 (42.4194, 2.6212) -> (43.1779, 2.6212)
  line L173 (43.1779, 2.6212) -> (43.1779, -3.6463)
  spline S168 degree 2 poles (46.246, -3.7484) (45.1666, -3.7484) (43.9802, -2.5377) (43.9802, -1.4194) knots 0 0 0 1 2 2 2
  spline S169 degree 2 poles (43.9802, -1.4194) (43.9802, -0.3205) (45.1326, 0.9826) (46.0612, 0.9826) knots 0 0 0 1 2 2 2
  spline S170 degree 2 poles (46.0612, 0.9826) (46.4794, 0.9826) (47.1261, 0.7395) (47.3643, 0.4818) knots 0 0 0 1 2 2 2
  spline S171 degree 2 poles (47.3643, 0.4818) (47.6074, 0.2241) (47.8651, -0.5199) (47.8651, -1.0596) knots 0 0 0 1 2 2 2
  line L174 (47.8651, -1.0596) -> (47.8651, -1.4729)
  line L175 (47.8651, -1.4729) -> (44.7484, -1.4729)
  spline S172 degree 2 poles (44.7484, -1.4729) (44.7484, -2.2557) (45.5361, -3.0871) (46.2363, -3.0871) knots 0 0 0 1 2 2 2
  spline S173 degree 2 poles (46.2363, -3.0871) (46.4843, -3.0871) (46.9656, -2.9753) (47.1601, -2.8878) knots 0 0 0 1 2 2 2
  spline S174 degree 2 poles (47.1601, -2.8878) (47.3643, -2.7905) (47.6463, -2.6203) (47.7387, -2.5425) knots 0 0 0 1 2 2 2
  line L176 (47.7387, -2.5425) -> (47.7825, -2.5425)
  line L177 (47.7825, -2.5425) -> (47.7825, -3.3691)
  spline S175 degree 2 poles (47.7825, -3.3691) (47.6512, -3.4226) (47.2525, -3.5782) (47.0969, -3.622) knots 0 0 0 1 2 2 2
  spline S176 degree 2 poles (47.0969, -3.622) (46.8781, -3.6852) (46.5183, -3.7484) (46.246, -3.7484) knots 0 0 0 1 2 2 2
  spline S177 degree 2 poles (47.1261, -0.8942) (47.1164, -0.5879) (46.9899, -0.1406) (46.8684, 0.0101) knots 0 0 0 1 2 2 2
  spline S178 degree 2 poles (46.8684, 0.0101) (46.7371, 0.1803) (46.3238, 0.3602) (46.0175, 0.3602) knots 0 0 0 1 2 2 2
  spline S179 degree 2 poles (46.0175, 0.3602) (45.716, 0.3602) (45.293, 0.1803) (45.118, 0.0053) knots 0 0 0 1 2 2 2
  spline S180 degree 2 poles (45.118, 0.0053) (44.9478, -0.1746) (44.7728, -0.6074) (44.7484, -0.8942) knots 0 0 0 1 2 2 2
  line L178 (44.7484, -0.8942) -> (47.1261, -0.8942)
  line L179 (51.9835, -3.6463) -> (51.2249, -3.6463)
  line L180 (51.2249, -3.6463) -> (51.2249, 0.8562)
  line L181 (51.2249, 0.8562) -> (51.9835, 0.8562)
  line L182 (51.9835, 0.8562) -> (51.9835, -3.6463)
  line L183 (52.0369, 1.6049) -> (51.1763, 1.6049)
  line L184 (51.1763, 1.6049) -> (51.1763, 2.3926)
  line L185 (51.1763, 2.3926) -> (52.0369, 2.3926)
  line L186 (52.0369, 2.3926) -> (52.0369, 1.6049)
  line L187 (56.6318, -3.6463) -> (55.8732, -3.6463)
  line L188 (55.8732, -3.6463) -> (55.8732, -1.079)
  spline S181 degree 2 poles (55.8732, -1.079) (55.8732, -0.7678) (55.8149, -0.233) (55.7274, -0.0725) knots 0 0 0 1 2 2 2
  spline S182 degree 2 poles (55.7274, -0.0725) (55.635, 0.0976) (55.3044, 0.263) (55.0224, 0.263) knots 0 0 0 1 2 2 2
  spline S183 degree 2 poles (55.0224, 0.263) (54.7403, 0.263) (54.1423, -0.0385) (53.8554, -0.2816) knots 0 0 0 1 2 2 2
  line L189 (53.8554, -0.2816) -> (53.8554, -3.6463)
  line L190 (53.8554, -3.6463) -> (53.0969, -3.6463)
  line L191 (53.0969, -3.6463) -> (53.0969, 0.8562)
  line L192 (53.0969, 0.8562) -> (53.8554, 0.8562)
  line L193 (53.8554, 0.8562) -> (53.8554, 0.3553)
  spline S184 degree 2 poles (53.8554, 0.3553) (54.1958, 0.6617) (54.8522, 0.9826) (55.2217, 0.9826) knots 0 0 0 1 2 2 2
  spline S185 degree 2 poles (55.2217, 0.9826) (55.883, 0.9826) (56.6318, 0.1074) (56.6318, -0.7241) knots 0 0 0 1 2 2 2
  line L194 (56.6318, -0.7241) -> (56.6318, -3.6463)
  point P0 (0, 0)
  constraints: 2 coincident, 4 other
extrude "Text" add sketch "Sketch1" along normal blind 1
body "Solid1"
